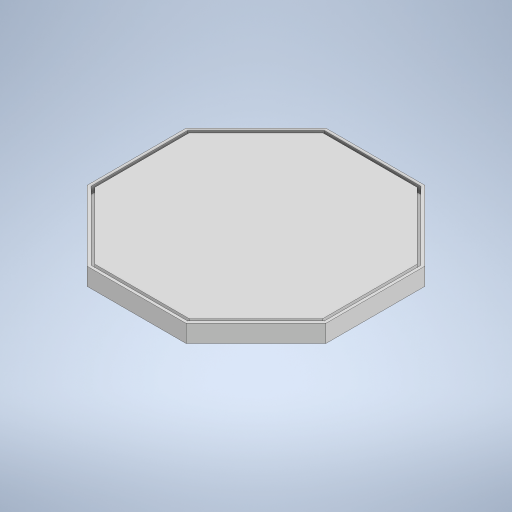
# Autodesk Inventor part: 팔각형 OV-PAM 상단
Saved by Autodesk Inventor 2024 (Build 280153000, 153)
## iProperties
Created: 2023-06-16
Part Number: 팔각형 OV-PAM 상단
Material: 일반
Document SubType Name: Modeling
Designer: jsw
Density: 1 g/cm^3
Appearance: 기본값
Author: jsw
Autodesk Inventor part; units mm, degrees
ref_plane "YZ Plane" through (0, 0, 0) normal (1, 0, 0) x (0, 1, 0)
ref_plane "XZ Plane" through (0, 0, 0) normal (0, 1, 0) x (-1, 0, 0)
ref_plane "XY Plane" through (0, 0, 0) normal (0, 0, 1) x (1, 0, 0)
sketch "스케치3" plane through (0, 0, 0) normal (0, 1, 0) x (-1, 0, 0)
  line L0 (34.1919, -14.1627) -> (14.1627, -34.1919)
  line L1 (14.1627, -34.1919) -> (-14.1627, -34.1919)
  line L2 (-14.1627, -34.1919) -> (-34.1919, -14.1627)
  line L3 (-34.1919, -14.1627) -> (-34.1919, 14.1627)
  line L4 (-34.1919, 14.1627) -> (-14.1627, 34.1919)
  line L5 (-14.1627, 34.1919) -> (14.1627, 34.1919)
  line L6 (14.1627, 34.1919) -> (34.1919, 14.1627)
  line L7 (34.1919, 14.1627) -> (34.1919, -14.1627)
  line L8 (13.5, -32.5919) -> (-13.5, -32.5919)
  line L9 (-13.5, -32.5919) -> (-32.5919, -13.5)
  line L10 (-32.5919, -13.5) -> (-32.5919, 13.5)
  line L11 (-32.5919, 13.5) -> (-13.5, 32.5919)
  line L12 (-13.5, 32.5919) -> (13.5, 32.5919)
  line L13 (13.5, 32.5919) -> (32.5919, 13.5)
  line L14 (32.5919, 13.5) -> (32.5919, -13.5)
  line L15 (32.5919, -13.5) -> (13.5, -32.5919)
  point P0 (0, 0)
  point P1 (0, 0)
  point P2 (0, 0)
  point P3 (0, 0)
  dimension "d66" = 27
  dimension "d67" = 1.6
  constraints: 32 end point, 3 coincident, 2 horizontal, 34 other
  measures "d66" distance of L8.start L8.end
  measures "d67" distance between parallel lines of L15 L0
extrude "돌출2" add sketch "스케치3" along normal blind 5 contours L0 L1 L2 L3 L4 L5 L6 L7 | L8 L9 L10 L11 L12 L13 L14 L15
sketch "스케치4" plane through (0, 5, 0) normal (0, 1, 0) x (1, 0, 0)
  line L0 (13.5, -32.5919) -> (-13.5, -32.5919)
  line L1 (-13.5, -32.5919) -> (-32.5919, -13.5)
  line L2 (-32.5919, -13.5) -> (-32.5919, 13.5)
  line L3 (-32.5919, 13.5) -> (-13.5, 32.5919)
  line L4 (-13.5, 32.5919) -> (13.5, 32.5919)
  line L5 (13.5, 32.5919) -> (32.5919, 13.5)
  line L6 (32.5919, 13.5) -> (32.5919, -13.5)
  line L7 (32.5919, -13.5) -> (13.5, -32.5919)
  line L8 (-13.8314, 33.3919) -> (13.8314, 33.3919)
  line L9 (13.8314, 33.3919) -> (33.3919, 13.8314)
  line L10 (33.3919, 13.8314) -> (33.3919, -13.8314)
  line L11 (33.3919, -13.8314) -> (13.8314, -33.3919)
  line L12 (13.8314, -33.3919) -> (-13.8314, -33.3919)
  line L13 (-13.8314, -33.3919) -> (-33.3919, -13.8314)
  line L14 (-33.3919, -13.8314) -> (-33.3919, 13.8314)
  line L15 (-33.3919, 13.8314) -> (-13.8314, 33.3919)
  point P0 (0, 0)
  point P1 (0, 0)
  point P2 (0, 0)
  dimension "d7" = 27
  dimension "d68" = 0.8
  constraints: 32 end point, 2 coincident, 2 horizontal, 34 other
  measures "d7" distance of L1.end L2.end
  measures "d68" distance between parallel lines of L3 L15
extrude "돌출3" cut sketch "스케치4" against normal blind 2
sketch "스케치9" plane through (0, 0, 0) normal (0, -1, 0) x (1, 0, 0)
  line L0 (7.5, 10) -> (2.5, 10)
  line L1 (2.5, 10) -> (2.5, -10)
  line L2 (2.5, -10) -> (7.5, -10)
  line L3 (7.5, -10) -> (7.5, 10)
  line L4 (7.5, 10) -> (2.5, -10) construction
  line L5 (2.5, 10) -> (7.5, -10) construction
  line L6 (-2.5, 10) -> (-7.5, 10)
  line L7 (-7.5, 10) -> (-7.5, -10)
  line L8 (-7.5, -10) -> (-2.5, -10)
  line L9 (-2.5, 10) -> (-7.5, -10) construction
  line L10 (-7.5, 10) -> (-2.5, -10) construction
  line L11 (-2.5, -10) -> (-2.5, 10)
  point P0 (0, 0)
  point P1 (5, 0)
  point P2 (-5, 0)
  dimension "d42" = 20
  dimension "d43" = 5
  dimension "d44" = 2.5
  dimension "d47" = 10
  constraints: 24 end point, 2 horizontal, 2 midpoint, 2 parallel, 1 collinear, 1 horizontal alignment, 1 perpendicular, 10 other
  measures "d42" distance of L2.end L0.start
  measures "d43" distance of L1.end L2.end
  measures "d44" distance from line of L1 point (0, 0)
  measures "d47" distance of L0.start L6.start
extrude "돌출8" add sketch "스케치9" along normal blind 10
sketch "스케치10" plane through (-7.5, 0, -10) normal (-1, 0, 0) x (0, 0, 1)
  circle A0 centre (15, -5) radius 1.25
  line L0 (19.9591, 0) -> (0.0886, 0)
  line L1 (24.1627, 0) -> (-4.1627, 0) projected
  circle A1 centre (5, -5) radius 1.25
  line L2 (20, 0) -> (20, -10) projected
  point P0 (10, 0)
  dimension "d54" = 2.5
  dimension "d57" = 10
  dimension "d62" = 5
  dimension "d63" = 5
  constraints: 2 centre point, 2 end point, 1 horizontal, 1 point on line, 2 other
  measures "d54" diameter of A0
  measures "d57" distance of A0.centre A1.centre
  measures "d62" distance from line of L0 A0.centre
  measures "d63" distance from line of L2 A0.centre
extrude "돌출9" cut sketch "스케치10" against normal blind 20
